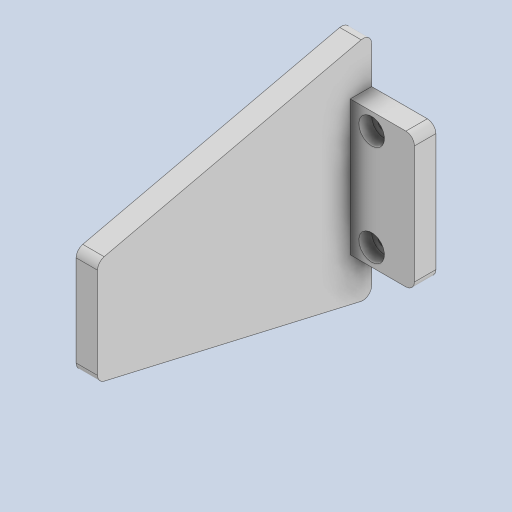
# Autodesk Inventor part: nail
Saved by Autodesk Inventor 2023 (Build 270158000, 158)
## iProperties
Created: 2024-12-14
Part Number: nail
Material: Generic
Document SubType Name: Modeling
Designer: kiyo
Density: 1 g/cm^3
Appearance: Default
Author: kiyo
Autodesk Inventor part; units mm, degrees
ref_plane "YZ Plane" through (0, 0, 0) normal (1, 0, 0) x (0, 1, 0)
ref_plane "XZ Plane" through (0, 0, 0) normal (0, 1, 0) x (-1, 0, 0)
ref_plane "XY Plane" through (0, 0, 0) normal (0, 0, 1) x (1, 0, 0)
sketch "スケッチ1" plane through (0, 0, 0) normal (0, 1, 0) x (-1, 0, 0)
  line L0 (0, 0) -> (0, 54)
  line L1 (0, 54) -> (-64, 39.2244)
  line L2 (-64, 39.2244) -> (-64, 14.7756)
  line L3 (-64, 14.7756) -> (0, 0)
  dimension "d0" = 77
  dimension "d1" = 77
  dimension "d2" = 64
  dimension "d3" = 54
  constraints: 8 end point, 2 vertical
  measures "d0" angle of L1 L0
  measures "d1" angle of L3 L0
  measures "d2" distance between parallel lines of L0 L2
  measures "d3" distance of L0.start L0.end
extrude "押し出し1" add sketch "スケッチ1" along normal blind 5
sketch "スケッチ2" plane through (0, 0, 0) normal (-1, 0, 0) x (0, 0, 1)
  line L0 (39.2244, 5) -> (14.7756, 5) projected
  line L1 (42.75, 5) -> (11.25, 5)
  line L2 (11.25, 5) -> (11.25, 20)
  line L3 (11.25, 20) -> (42.75, 20)
  line L4 (42.75, 20) -> (42.75, 5)
  line L5 (54, 0) -> (54, 5) projected
  point P0 (0, 0)
  dimension "d6" = 31.5
  dimension "d7" = 15
  dimension "d8" = 11.25
  constraints: 8 end point, 2 parallel, 1 horizontal, 1 perpendicular, 1 point on line
  measures "d6" distance of L2.end L3.end
  measures "d7" distance of L1.end L2.end
  measures "d8" distance between parallel lines of L4 L5
extrude "押し出し2" add sketch "スケッチ2" against normal blind 5
sketch "スケッチ3" plane through (5, 0, 0) normal (1, 0, 0) x (0, 0, -1)
  line L0 (-42.75, 20) -> (-42.75, 5) projected
  line L1 (-39.2244, 5) -> (-14.7756, 5) projected
  point P0 (0, 0)
  point P1 (-38.75, 10)
  point P2 (-15.25, 10)
  dimension "d15" = 10
  dimension "d11" = 4
  dimension "d12" = 5
  dimension "d18" = 23.5
  constraints: 1 horizontal, 1 vertical, 1 other
  measures "d11" distance from line of L0 point (-38.75, 10)
  measures "d12" distance from line of L1 point (-38.75, 10)
  measures "d18" distance of point (-38.75, 10) point (-15.25, 10)
hole "穴1" at (5, 10, 38.75) at (5, 10, 15.25) direction (-1, 0, 0) diameter 3.2 depth 8 tip angle 118 counterbore diameter 6 counterbore depth 3
fillet "フィレット1" radius 2 6 edges at (0, 2.5, 54) (0, 2.5, 0) (64, 2.5, 14.7756) (64, 2.5, 39.2244) (2.5, 20, 42.75) (2.5, 20, 11.25)
equation "\"d1\" = d0"
